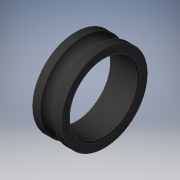
# Autodesk Inventor part: 60/28 Inner Ring
Saved by Autodesk Inventor 2019 (Build 230136000, 136)
## iProperties
Created: 2024-02-20
Part Number: 60/28 Inner Ring
Material: Generic
Catalog Web Link: www.cadenas.de
Description: Open type ir-Deep Groove Ball Bearings
Vendor: NTN
Document SubType Name: Modeling
Designer: psAdmin
Manufacturer: NTN
Mass: 3.96718 g
Surface Area: 31.8697 cm^2
Volume: 3.96718 cm^3
Density: 1 g/cm^3
Appearance: PSOLRGB-175-175-175
Category: PARTsolutions
Company: NTN
Title: 60/28 Inner Ring
Author: Cadenas PARTsolutions
Comments: Deep Groove Ball Bearings
PSOL_IDENT_0: {$CADENAS_DATA/23d-libs/ntn/ball_roller_bearings/deep_groove_bb/deep_groove_bb/6_types/dgbb_ir.prj},
PSOL_IDENT_1: 179 {VTYP=3D},{NB=60/28 Inner Ring},{LINA=60/28 Inner Ring},{NN=Open type ir},{DATE=17.10.2023 22:55
PSOL_IDENT_2: :17},{GEOMDATE=11.08.2020 08:58:19},{VERSION=},{LINEID=480},{WBVAR=},{WBNUMERIC=}  {NB=60/28 Inner R
PSOL_IDENT_3: ing},{LINA=60/28 Inner Ring},{KT=DUMMY},{IDNR=},{SD=28},{D=52},{B=12},{R=0.6},{ORDER1=60/28},{ORDER=
PSOL_IDENT_4: 60/28},{VERS=1},{CR=12.5},{COR=7.40},{CRF=1270},{CORF=755},{LSG=14000},{LSO=16000},{MASS=0.10},{RNS=
PSOL_IDENT_5: 0.5},{LLH=10000},{LLU=8400},{ST=ZZ},{NCST=LLB},{LTST=LLH},{CST=LLU},{SRG=N},{SR=NR},{D1=49.73},{A=2.
PSOL_IDENT_6: 06},{BA=1.35},{R0=0.40},{D2=57.9},{F=1.12},{DA1=32},{DA2=34},{DA=48},{DX=58.5},{CY=2.9},{CZ=1.2},{RA
PSOL_IDENT_7: S=0.6},{RNAS=0.5},{X=12},{XVE=2}
NB: 60/28 Inner Ring
NN: Open type ir
NT: Deep Groove Ball Bearings
NBSYN: $ORDER. Inner Ring
LINA: 60/28 Inner Ring
CATALOG: NTN Corporation
SD: 28
D: 52
B: 12
R: 0.6
ORDER1: 60/28
ORDER: 60/28
VERS: 1
CR: 12.5
COR: 7.40
CRF: 1270
CORF: 755
LSG: 14000
LSO: 16000
MASS: 0.10
RNS: 0.5
LLH: 10000
LLU: 8400
ST: ZZ
NCST: LLB
LTST: LLH
CST: LLU
SRG: N
SR: NR
D1: 49.73
A: 2.06
BA: 1.35
R0: 0.4
D2: 57.9
F: 1.12
DA1: 32
DA2: 34
DA: 48
DX: 58.5
CY: 2.9
CZ: 1.2
RAS: 0.6
RNAS: 0.5
XVE: 2
SUPPLIER: NTN
ARTICLENO: 60/28 Inner Ring
BOMINFO: 60/28 Inner Ring
CREATOR: CADENAS GmbH
Autodesk Inventor part; units mm, degrees
sketch "Sketch_1" plane through (0, 0, 0) normal (0, 0, 1) x (1, 0, 0)
  line L0 (12, 0) -> (0, 0)
  arc A0 (0, 14.6) -> (0.6, 14) centre (0.6, 14.6) ccw
  line L1 (0.6, 14) -> (11.4, 14)
  arc A1 (11.4, 14) -> (12, 14.6) centre (11.4, 14.6) ccw
  line L2 (12, 14.6) -> (12, 17.84)
  line L3 (12, 17.84) -> (8.88, 17.84)
  arc A2 (3.12, 17.84) -> (8.88, 17.84) centre (6, 20) ccw
  line L4 (3.12, 17.84) -> (0, 17.84)
  line L5 (0, 17.84) -> (0, 14.6)
  constraints: 12 end point, 6 point on circle, 3 centre point
revolve "Revolution1" add sketch "Sketch_1" angle 360 about axis through (12, 0, 0) along (1, 0, 0)
ref_plane "dgbb_ir_XY" through (0, 0, 0) normal (1, 0, 0) x (0, 0, -1)
ref_plane "dgbb_ir_YZ" through (0, 0, 0) normal (0, 0, -1) x (0, 1, 0)
ref_plane "dgbb_ir_ZX" through (0, 0, 0) normal (0, 1, 0) x (1, 0, 0)
body "Solid1"
